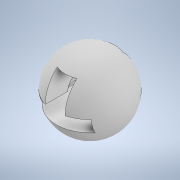
# Autodesk Inventor part: 1_2
Saved by Autodesk Inventor 2020.1 (Build 241239000, 239)
## iProperties
Created: 2022-02-16
Part Number: 1_2
Material: Типовые
Document SubType Name: Modeling
Designer: User
Density: 1 g/cm^3
Appearance: По умолчанию
Author: User
Autodesk Inventor part; units mm, degrees
ref_plane "YZ Plane" through (0, 0, 0) normal (1, 0, 0) x (0, 1, 0)
ref_plane "XZ Plane" through (0, 0, 0) normal (0, 1, 0) x (-1, 0, 0)
ref_plane "XY Plane" through (0, 0, 0) normal (0, 0, 1) x (1, 0, 0)
sketch "Эскиз1" plane through (0, 0, 0) normal (0, 0, 1) x (1, 0, 0)
  circle A0 centre (0, 0) radius 55
  circle A1 centre (0, 0) radius 24
  line L0 (0, -55) -> (0, 55)
  point P0 (0, 24)
  point P1 (0, -24)
  dimension "d0" = 110
  dimension "d1" = 48
  constraints: 2 centre point, 2 coincident, 2 end point, 2 point on circle, 1 vertical
  measures "d0" diameter of A0
  measures "d1" diameter of A1
revolve "Вращение1" add sketch "Эскиз1" angle 360 about axis through (0, -55, 0) along (0, 1, 0) picked at (-44.4519, -0.9643) contours L0 A1 A0
sketch "Эскиз2" plane through (0, 0, 0) normal (0, 0, 1) x (1, 0, 0)
  line L0 (15, 0) -> (-15, 0)
  line L1 (-15, 0) -> (-15, 40)
  line L2 (-15, 40) -> (15, 40)
  line L3 (15, 40) -> (15, 0)
  line L4 (-40, 0) -> (40, 0)
  line L5 (40, 0) -> (40, -20)
  line L6 (40, -20) -> (-40, -20)
  line L7 (-40, -20) -> (-40, 0)
  point P0 (0, 0)
  point P1 (0, 0)
  point P2 (0, 0)
  point P3 (0, 0)
  dimension "d3" = 0
  dimension "d4" = 0
  dimension "d5" = 80
  dimension "d6" = 20
  dimension "d7" = 30
  dimension "d8" = 60
  constraints: 16 end point, 4 parallel, 2 horizontal, 2 midpoint, 2 perpendicular, 1 coincident
  measures "d3" distance of point (0, 0) point (0, 0)
  measures "d4" distance of point (0, 0) point (0, 0)
  measures "d5" distance of L5.end L6.end
  measures "d6" distance of L6.end L4.start
  measures "d7" distance of L1.end L2.end
  measures "d8" vertical distance of L2.end L5.end
extrude "Выдавливание1" cut sketch "Эскиз2" against normal mid plane 1000
